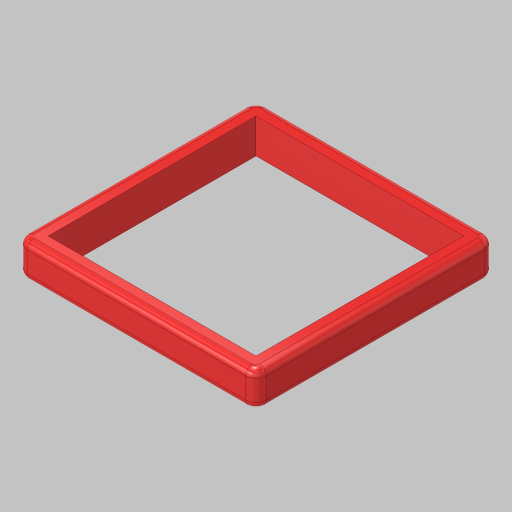
# Autodesk Inventor part: BP-0036
Saved by Autodesk Inventor 2023.5 (Build 275446000, 446)
## iProperties
Created: 2025-01-26
Part Number: BP-0036
Material: Fabric
Document SubType Name: Modeling
Designer: slick
Surface Area: 10712.9 cm^2
Volume: 20408 cm^3
Appearance: Light Red
Author: slick
Autodesk Inventor part; units mm, degrees
ref_plane "YZ Plane" through (0, 0, 0) normal (1, 0, 0) x (0, 1, 0)
ref_plane "XZ Plane" through (0, 0, 0) normal (0, 1, 0) x (-1, 0, 0)
ref_plane "XY Plane" through (0, 0, 0) normal (0, 0, 1) x (1, 0, 0)
sketch "Sketch1" plane through (0, 0, 0) normal (0, 1, 0) x (-1, 0, 0)
  line L0 (-381, -381) -> (381, -381)
  line L1 (381, -381) -> (381, 381)
  line L2 (381, 381) -> (-381, 381)
  line L3 (-381, 381) -> (-381, -381)
  line L4 (-381, -381) -> (381, 381) construction
  line L5 (381, -381) -> (-381, 381) construction
  line L6 (438.15, 438.15) -> (438.15, -438.15)
  line L7 (438.15, -438.15) -> (-438.15, -438.15)
  line L8 (-438.15, -438.15) -> (-438.15, 438.15)
  line L9 (-438.15, 438.15) -> (438.15, 438.15)
  point P0 (0, 0)
  dimension "d0" = 762
  dimension "d1" = 762
  dimension "d2" = 57.15
  constraints: 20 end point, 4 parallel, 2 midpoint, 2 perpendicular, 1 horizontal, 3 other
  measures "d0" distance of L2.end L1.end
  measures "d1" distance of L1.end L0.end
  measures "d2" distance between parallel lines of L1 L6
extrude "Extrusion1" add sketch "Sketch1" along normal blind 127
fillet "Fillet1" radius 38.1 4 edges at (-438.15, 63.5, 438.15) (438.15, 63.5, 438.15) (438.15, 63.5, -438.15) (-438.15, 63.5, -438.15)
fillet "Fillet2" radius 25.4 16 edges at (426.9908, 127, 426.9908) (438.15, 127, 0) (426.9908, 127, -426.9908) (0, 127, -438.15) (-426.9908, 127, -426.9908) (-438.15, 127, 0) (-426.9908, 127, 426.9908) (0, 127, 438.15) (426.9908, 0, 426.9908) (438.15, 0, 0) (426.9908, 0, -426.9908) (0, 0, -438.15) (-426.9908, 0, -426.9908) (-438.15, 0, 0) (-426.9908, 0, 426.9908) (0, 0, 438.15)
body "Solid1"
